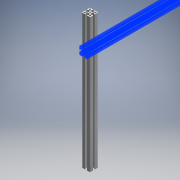
# Autodesk Inventor part: Propile_500
Saved by Autodesk Inventor 2019 (Build 230136000, 136)
## iProperties
Created: 2019-04-24
Part Number: Propile_500
Material: 알루미늄 6061
Document SubType Name: Modeling
Designer: hinmo
Density: 2.7 g/cm^3
Appearance: 알루미늄 - 평지
Mass: 433.812 g
Surface Area: 1856.02 cm^2
Volume: 160.671 cm^3
Author: hinmo
Autodesk Inventor part; units mm, degrees
ref_plane "YZ Plane" through (0, 0, 0) normal (1, 0, 0) x (0, 1, 0)
ref_plane "XZ Plane" through (0, 0, 0) normal (0, 1, 0) x (-1, 0, 0)
ref_plane "XY Plane" through (0, 0, 0) normal (0, 0, 1) x (1, 0, 0)
sketch "스케치1" plane through (0, 0, 0) normal (0, 1, 0) x (-1, 0, 0)
  arc A0 (556.3252, 935.7031) -> (557.3252, 936.7031) centre (556.3252, 936.7031) ccw projected
  line L0 (557.3252, 936.7031) -> (557.3252, 938.2031) projected
  line L1 (557.3252, 938.2031) -> (555.3752, 938.2031) projected
  line L2 (555.3752, 938.2031) -> (554.3965, 941.8963) projected
  arc A1 (557.0402, 946.2031) -> (554.3965, 941.8963) centre (561.0724, 940.7632) ccw projected
  line L3 (557.0402, 946.2031) -> (559.9752, 946.2031) projected
  line L4 (559.9752, 946.2031) -> (560.4752, 946.7031) projected
  line L5 (560.4752, 946.7031) -> (560.9752, 946.2031) projected
  line L6 (560.9752, 946.2031) -> (563.9102, 946.2031) projected
  arc A2 (566.5539, 941.8963) -> (563.9102, 946.2031) centre (559.878, 940.7632) ccw projected
  line L7 (566.5539, 941.8963) -> (565.5752, 938.2031) projected
  line L8 (565.5752, 938.2031) -> (563.6252, 938.2031) projected
  line L9 (563.6252, 938.2031) -> (563.6252, 936.7031) projected
  arc A3 (563.6252, 936.7031) -> (564.6252, 935.7031) centre (564.6252, 936.7031) ccw projected
  line L10 (564.6252, 935.7031) -> (573.9752, 935.7031) projected
  arc A4 (573.9752, 935.7031) -> (575.4752, 937.2031) centre (573.9752, 937.2031) ccw projected
  line L11 (575.4752, 937.2031) -> (575.4752, 946.5531) projected
  arc A5 (575.4752, 946.5531) -> (574.4752, 947.5531) centre (574.4752, 946.5531) ccw projected
  line L12 (574.4752, 947.5531) -> (572.9752, 947.5531) projected
  line L13 (572.9752, 947.5531) -> (572.9752, 945.6031) projected
  line L14 (572.9752, 945.6031) -> (569.282, 944.6244) projected
  arc A6 (564.9752, 947.2681) -> (569.282, 944.6244) centre (570.4151, 951.3003) ccw projected
  line L15 (564.9752, 947.2681) -> (564.9752, 950.2031) projected
  line L16 (564.9752, 950.2031) -> (564.4752, 950.7031) projected
  line L17 (564.4752, 950.7031) -> (564.9752, 951.2031) projected
  line L18 (564.9752, 951.2031) -> (564.9752, 954.1381) projected
  arc A7 (569.282, 956.7818) -> (564.9752, 954.1381) centre (570.4151, 950.1059) ccw projected
  line L19 (569.282, 956.7818) -> (572.9752, 955.8031) projected
  line L20 (572.9752, 955.8031) -> (572.9752, 953.8531) projected
  line L21 (572.9752, 953.8531) -> (574.4752, 953.8531) projected
  arc A8 (574.4752, 953.8531) -> (575.4752, 954.8531) centre (574.4752, 954.8531) ccw projected
  line L22 (575.4752, 954.8531) -> (575.4752, 964.2031) projected
  arc A9 (575.4752, 964.2031) -> (573.9752, 965.7031) centre (573.9752, 964.2031) ccw projected
  line L23 (573.9752, 965.7031) -> (564.6252, 965.7031) projected
  arc A10 (564.6252, 965.7031) -> (563.6252, 964.7031) centre (564.6252, 964.7031) ccw projected
  line L24 (563.6252, 964.7031) -> (563.6252, 963.2031) projected
  line L25 (563.6252, 963.2031) -> (565.5752, 963.2031) projected
  line L26 (565.5752, 963.2031) -> (566.5539, 959.51) projected
  arc A11 (563.9102, 955.2031) -> (566.5539, 959.51) centre (559.878, 960.6431) ccw projected
  line L27 (563.9102, 955.2031) -> (560.9752, 955.2031) projected
  line L28 (560.9752, 955.2031) -> (560.4752, 954.7031) projected
  line L29 (560.4752, 954.7031) -> (559.9752, 955.2031) projected
  line L30 (559.9752, 955.2031) -> (557.0402, 955.2031) projected
  arc A12 (554.3965, 959.51) -> (557.0402, 955.2031) centre (561.0724, 960.6431) ccw projected
  line L31 (554.3965, 959.51) -> (555.3752, 963.2031) projected
  line L32 (555.3752, 963.2031) -> (557.3252, 963.2031) projected
  line L33 (557.3252, 963.2031) -> (557.3252, 964.7031) projected
  arc A13 (557.3252, 964.7031) -> (556.3252, 965.7031) centre (556.3252, 964.7031) ccw projected
  line L34 (556.3252, 965.7031) -> (546.9752, 965.7031) projected
  arc A14 (546.9752, 965.7031) -> (545.4752, 964.2031) centre (546.9752, 964.2031) ccw projected
  line L35 (545.4752, 964.2031) -> (545.4752, 954.8531) projected
  arc A15 (545.4752, 954.8531) -> (546.4752, 953.8531) centre (546.4752, 954.8531) ccw projected
  line L36 (546.4752, 953.8531) -> (547.9752, 953.8531) projected
  line L37 (547.9752, 953.8531) -> (547.9752, 955.8031) projected
  line L38 (547.9752, 955.8031) -> (551.6683, 956.7818) projected
  arc A16 (555.9752, 954.1381) -> (551.6683, 956.7818) centre (550.5352, 950.1059) ccw projected
  line L39 (555.9752, 954.1381) -> (555.9752, 951.2031) projected
  line L40 (555.9752, 951.2031) -> (556.4752, 950.7031) projected
  line L41 (556.4752, 950.7031) -> (555.9752, 950.2031) projected
  line L42 (555.9752, 950.2031) -> (555.9752, 947.2681) projected
  arc A17 (551.6683, 944.6244) -> (555.9752, 947.2681) centre (550.5352, 951.3003) ccw projected
  line L43 (551.6683, 944.6244) -> (547.9752, 945.6031) projected
  line L44 (547.9752, 945.6031) -> (547.9752, 947.5531) projected
  line L45 (547.9752, 947.5531) -> (546.4752, 947.5531) projected
  arc A18 (546.4752, 947.5531) -> (545.4752, 946.5531) centre (546.4752, 946.5531) ccw projected
  line L46 (545.4752, 946.5531) -> (545.4752, 937.2031) projected
  arc A19 (545.4752, 937.2031) -> (546.9752, 935.7031) centre (546.9752, 937.2031) ccw projected
  line L47 (546.9752, 935.7031) -> (556.3252, 935.7031) projected
  arc A20 (573.0595, 959.1795) -> (573.0595, 962.2268) centre (570.4752, 960.7031) ccw projected
  line L48 (573.0595, 959.1795) -> (574.0055, 958.2335) projected
  line L49 (574.0055, 958.2335) -> (572.9448, 957.1728) projected
  line L50 (572.9448, 957.1728) -> (571.9988, 958.1188) projected
  arc A21 (568.9515, 958.1188) -> (571.9988, 958.1188) centre (570.4752, 960.7031) ccw projected
  line L51 (568.9515, 958.1188) -> (568.0055, 957.1728) projected
  line L52 (568.0055, 957.1728) -> (566.9448, 958.2335) projected
  line L53 (566.9448, 958.2335) -> (567.8909, 959.1795) projected
  arc A22 (567.8909, 962.2268) -> (567.8909, 959.1795) centre (570.4752, 960.7031) ccw projected
  line L54 (567.8909, 962.2268) -> (566.9448, 963.1728) projected
  line L55 (566.9448, 963.1728) -> (568.0055, 964.2335) projected
  line L56 (568.0055, 964.2335) -> (568.9515, 963.2874) projected
  arc A23 (571.9988, 963.2874) -> (568.9515, 963.2874) centre (570.4752, 960.7031) ccw projected
  line L57 (571.9988, 963.2874) -> (572.9448, 964.2335) projected
  line L58 (572.9448, 964.2335) -> (574.0055, 963.1728) projected
  line L59 (574.0055, 963.1728) -> (573.0595, 962.2268) projected
  line L60 (563.5055, 952.6728) -> (562.5713, 952.0656) projected
  arc A24 (562.5713, 949.3407) -> (562.5713, 952.0656) centre (560.4752, 950.7031) ccw projected
  line L61 (562.5713, 949.3407) -> (563.5055, 948.7335) projected
  line L62 (563.5055, 948.7335) -> (562.4448, 947.6728) projected
  line L63 (562.4448, 947.6728) -> (561.8376, 948.607) projected
  arc A25 (559.1127, 948.607) -> (561.8376, 948.607) centre (560.4752, 950.7031) ccw projected
  line L64 (559.1127, 948.607) -> (558.5055, 947.6728) projected
  line L65 (558.5055, 947.6728) -> (557.4448, 948.7335) projected
  line L66 (557.4448, 948.7335) -> (558.3791, 949.3407) projected
  arc A26 (558.3791, 952.0656) -> (558.3791, 949.3407) centre (560.4752, 950.7031) ccw projected
  line L67 (558.3791, 952.0656) -> (557.4448, 952.6728) projected
  line L68 (557.4448, 952.6728) -> (558.5055, 953.7335) projected
  line L69 (558.5055, 953.7335) -> (559.1127, 952.7992) projected
  arc A27 (561.8376, 952.7992) -> (559.1127, 952.7992) centre (560.4752, 950.7031) ccw projected
  line L70 (561.8376, 952.7992) -> (562.4448, 953.7335) projected
  line L71 (562.4448, 953.7335) -> (563.5055, 952.6728) projected
  arc A28 (571.9988, 943.2874) -> (568.9515, 943.2874) centre (570.4752, 940.7031) ccw projected
  line L72 (571.9988, 943.2874) -> (572.9448, 944.2335) projected
  line L73 (572.9448, 944.2335) -> (574.0055, 943.1728) projected
  line L74 (574.0055, 943.1728) -> (573.0595, 942.2268) projected
  arc A29 (573.0595, 939.1795) -> (573.0595, 942.2268) centre (570.4752, 940.7031) ccw projected
  line L75 (573.0595, 939.1795) -> (574.0055, 938.2335) projected
  line L76 (574.0055, 938.2335) -> (572.9448, 937.1728) projected
  line L77 (572.9448, 937.1728) -> (571.9988, 938.1188) projected
  arc A30 (568.9515, 938.1188) -> (571.9988, 938.1188) centre (570.4752, 940.7031) ccw projected
  line L78 (568.9515, 938.1188) -> (568.0055, 937.1728) projected
  line L79 (568.0055, 937.1728) -> (566.9448, 938.2335) projected
  line L80 (566.9448, 938.2335) -> (567.8909, 939.1795) projected
  arc A31 (567.8909, 942.2268) -> (567.8909, 939.1795) centre (570.4752, 940.7031) ccw projected
  line L81 (567.8909, 942.2268) -> (566.9448, 943.1728) projected
  line L82 (566.9448, 943.1728) -> (568.0055, 944.2335) projected
  line L83 (568.0055, 944.2335) -> (568.9515, 943.2874) projected
  arc A32 (548.9515, 958.1188) -> (551.9988, 958.1188) centre (550.4752, 960.7031) ccw projected
  line L84 (548.9515, 958.1188) -> (548.0055, 957.1728) projected
  line L85 (548.0055, 957.1728) -> (546.9448, 958.2335) projected
  line L86 (546.9448, 958.2335) -> (547.8909, 959.1795) projected
  arc A33 (547.8909, 962.2268) -> (547.8909, 959.1795) centre (550.4752, 960.7031) ccw projected
  line L87 (547.8909, 962.2268) -> (546.9448, 963.1728) projected
  line L88 (546.9448, 963.1728) -> (548.0055, 964.2335) projected
  line L89 (548.0055, 964.2335) -> (548.9515, 963.2874) projected
  arc A34 (551.9988, 963.2874) -> (548.9515, 963.2874) centre (550.4752, 960.7031) ccw projected
  line L90 (551.9988, 963.2874) -> (552.9448, 964.2335) projected
  line L91 (552.9448, 964.2335) -> (554.0055, 963.1728) projected
  line L92 (554.0055, 963.1728) -> (553.0595, 962.2268) projected
  arc A35 (553.0595, 959.1795) -> (553.0595, 962.2268) centre (550.4752, 960.7031) ccw projected
  line L93 (553.0595, 959.1795) -> (554.0055, 958.2335) projected
  line L94 (554.0055, 958.2335) -> (552.9448, 957.1728) projected
  line L95 (552.9448, 957.1728) -> (551.9988, 958.1188) projected
  arc A36 (553.0595, 939.1795) -> (553.0595, 942.2268) centre (550.4752, 940.7031) ccw projected
  line L96 (553.0595, 939.1795) -> (554.0055, 938.2335) projected
  line L97 (554.0055, 938.2335) -> (552.9448, 937.1728) projected
  line L98 (552.9448, 937.1728) -> (551.9988, 938.1188) projected
  arc A37 (548.9515, 938.1188) -> (551.9988, 938.1188) centre (550.4752, 940.7031) ccw projected
  line L99 (548.9515, 938.1188) -> (548.0055, 937.1728) projected
  line L100 (548.0055, 937.1728) -> (546.9448, 938.2335) projected
  line L101 (546.9448, 938.2335) -> (547.8909, 939.1795) projected
  arc A38 (547.8909, 942.2268) -> (547.8909, 939.1795) centre (550.4752, 940.7031) ccw projected
  line L102 (547.8909, 942.2268) -> (546.9448, 943.1728) projected
  line L103 (546.9448, 943.1728) -> (548.0055, 944.2335) projected
  line L104 (548.0055, 944.2335) -> (548.9515, 943.2874) projected
  arc A39 (551.9988, 943.2874) -> (548.9515, 943.2874) centre (550.4752, 940.7031) ccw projected
  line L105 (551.9988, 943.2874) -> (552.9448, 944.2335) projected
  line L106 (552.9448, 944.2335) -> (554.0055, 943.1728) projected
  line L107 (554.0055, 943.1728) -> (553.0595, 942.2268) projected
  arc A40 (-4.15, -15) -> (-3.15, -14) centre (-4.15, -14) ccw
  line L108 (-3.15, -14) -> (-3.15, -12.5)
  line L109 (-3.15, -12.5) -> (-5.1, -12.5)
  line L110 (-5.1, -12.5) -> (-6.0787, -8.8068)
  arc A41 (-3.435, -4.5) -> (-6.0787, -8.8068) centre (0.5972, -9.94) ccw
  line L111 (-3.435, -4.5) -> (-0.5, -4.5)
  line L112 (-0.5, -4.5) -> (0, -4)
  line L113 (0, -4) -> (0.5, -4.5)
  line L114 (0.5, -4.5) -> (3.435, -4.5)
  arc A42 (6.0787, -8.8068) -> (3.435, -4.5) centre (-0.5972, -9.94) ccw
  line L115 (6.0787, -8.8068) -> (5.1, -12.5)
  line L116 (5.1, -12.5) -> (3.15, -12.5)
  line L117 (3.15, -12.5) -> (3.15, -14)
  arc A43 (3.15, -14) -> (4.15, -15) centre (4.15, -14) ccw
  line L118 (4.15, -15) -> (13.5, -15)
  arc A44 (13.5, -15) -> (15, -13.5) centre (13.5, -13.5) ccw
  line L119 (15, -13.5) -> (15, -4.15)
  arc A45 (15, -4.15) -> (14, -3.15) centre (14, -4.15) ccw
  line L120 (14, -3.15) -> (12.5, -3.15)
  line L121 (12.5, -3.15) -> (12.5, -5.1)
  line L122 (12.5, -5.1) -> (8.8068, -6.0787)
  arc A46 (4.5, -3.435) -> (8.8068, -6.0787) centre (9.94, 0.5972) ccw
  line L123 (4.5, -3.435) -> (4.5, -0.5)
  line L124 (4.5, -0.5) -> (4, 0)
  line L125 (4, 0) -> (4.5, 0.5)
  line L126 (4.5, 0.5) -> (4.5, 3.435)
  arc A47 (8.8068, 6.0787) -> (4.5, 3.435) centre (9.94, -0.5972) ccw
  line L127 (8.8068, 6.0787) -> (12.5, 5.1)
  line L128 (12.5, 5.1) -> (12.5, 3.15)
  line L129 (12.5, 3.15) -> (14, 3.15)
  arc A48 (14, 3.15) -> (15, 4.15) centre (14, 4.15) ccw
  line L130 (15, 4.15) -> (15, 13.5)
  arc A49 (15, 13.5) -> (13.5, 15) centre (13.5, 13.5) ccw
  line L131 (13.5, 15) -> (4.15, 15)
  arc A50 (4.15, 15) -> (3.15, 14) centre (4.15, 14) ccw
  line L132 (3.15, 14) -> (3.15, 12.5)
  line L133 (3.15, 12.5) -> (5.1, 12.5)
  line L134 (5.1, 12.5) -> (6.0787, 8.8068)
  arc A51 (3.435, 4.5) -> (6.0787, 8.8068) centre (-0.5972, 9.94) ccw
  line L135 (3.435, 4.5) -> (0.5, 4.5)
  line L136 (0.5, 4.5) -> (0, 4)
  line L137 (0, 4) -> (-0.5, 4.5)
  line L138 (-0.5, 4.5) -> (-3.435, 4.5)
  arc A52 (-6.0787, 8.8068) -> (-3.435, 4.5) centre (0.5972, 9.94) ccw
  line L139 (-6.0787, 8.8068) -> (-5.1, 12.5)
  line L140 (-5.1, 12.5) -> (-3.15, 12.5)
  line L141 (-3.15, 12.5) -> (-3.15, 14)
  arc A53 (-3.15, 14) -> (-4.15, 15) centre (-4.15, 14) ccw
  line L142 (-4.15, 15) -> (-13.5, 15)
  arc A54 (-13.5, 15) -> (-15, 13.5) centre (-13.5, 13.5) ccw
  line L143 (-15, 13.5) -> (-15, 4.15)
  arc A55 (-15, 4.15) -> (-14, 3.15) centre (-14, 4.15) ccw
  line L144 (-14, 3.15) -> (-12.5, 3.15)
  line L145 (-12.5, 3.15) -> (-12.5, 5.1)
  line L146 (-12.5, 5.1) -> (-8.8068, 6.0787)
  arc A56 (-4.5, 3.435) -> (-8.8068, 6.0787) centre (-9.94, -0.5972) ccw
  line L147 (-4.5, 3.435) -> (-4.5, 0.5)
  line L148 (-4.5, 0.5) -> (-4, 0)
  line L149 (-4, 0) -> (-4.5, -0.5)
  line L150 (-4.5, -0.5) -> (-4.5, -3.435)
  arc A57 (-8.8068, -6.0787) -> (-4.5, -3.435) centre (-9.94, 0.5972) ccw
  line L151 (-8.8068, -6.0787) -> (-12.5, -5.1)
  line L152 (-12.5, -5.1) -> (-12.5, -3.15)
  line L153 (-12.5, -3.15) -> (-14, -3.15)
  arc A58 (-14, -3.15) -> (-15, -4.15) centre (-14, -4.15) ccw
  line L154 (-15, -4.15) -> (-15, -13.5)
  arc A59 (-15, -13.5) -> (-13.5, -15) centre (-13.5, -13.5) ccw
  line L155 (-13.5, -15) -> (-4.15, -15)
  arc A60 (12.5843, 8.4764) -> (12.5843, 11.5236) centre (10, 10) ccw
  line L156 (12.5843, 8.4764) -> (13.5303, 7.5303)
  line L157 (13.5303, 7.5303) -> (12.4697, 6.4697)
  line L158 (12.4697, 6.4697) -> (11.5236, 7.4157)
  arc A61 (8.4764, 7.4157) -> (11.5236, 7.4157) centre (10, 10) ccw
  line L159 (8.4764, 7.4157) -> (7.5303, 6.4697)
  line L160 (7.5303, 6.4697) -> (6.4697, 7.5303)
  line L161 (6.4697, 7.5303) -> (7.4157, 8.4764)
  arc A62 (7.4157, 11.5236) -> (7.4157, 8.4764) centre (10, 10) ccw
  line L162 (7.4157, 11.5236) -> (6.4697, 12.4697)
  line L163 (6.4697, 12.4697) -> (7.5303, 13.5303)
  line L164 (7.5303, 13.5303) -> (8.4764, 12.5843)
  arc A63 (11.5236, 12.5843) -> (8.4764, 12.5843) centre (10, 10) ccw
  line L165 (11.5236, 12.5843) -> (12.4697, 13.5303)
  line L166 (12.4697, 13.5303) -> (13.5303, 12.4697)
  line L167 (13.5303, 12.4697) -> (12.5843, 11.5236)
  line L168 (3.0303, 1.9697) -> (2.0961, 1.3624)
  arc A64 (2.0961, -1.3624) -> (2.0961, 1.3624) centre (0, 0) ccw
  line L169 (2.0961, -1.3624) -> (3.0303, -1.9697)
  line L170 (3.0303, -1.9697) -> (1.9697, -3.0303)
  line L171 (1.9697, -3.0303) -> (1.3624, -2.0961)
  arc A65 (-1.3624, -2.0961) -> (1.3624, -2.0961) centre (0, 0) ccw
  line L172 (-1.3624, -2.0961) -> (-1.9697, -3.0303)
  line L173 (-1.9697, -3.0303) -> (-3.0303, -1.9697)
  line L174 (-3.0303, -1.9697) -> (-2.0961, -1.3624)
  arc A66 (-2.0961, 1.3624) -> (-2.0961, -1.3624) centre (0, 0) ccw
  line L175 (-2.0961, 1.3624) -> (-3.0303, 1.9697)
  line L176 (-3.0303, 1.9697) -> (-1.9697, 3.0303)
  line L177 (-1.9697, 3.0303) -> (-1.3624, 2.0961)
  arc A67 (1.3624, 2.0961) -> (-1.3624, 2.0961) centre (0, 0) ccw
  line L178 (1.3624, 2.0961) -> (1.9697, 3.0303)
  line L179 (1.9697, 3.0303) -> (3.0303, 1.9697)
  arc A68 (11.5236, -7.4157) -> (8.4764, -7.4157) centre (10, -10) ccw
  line L180 (11.5236, -7.4157) -> (12.4697, -6.4697)
  line L181 (12.4697, -6.4697) -> (13.5303, -7.5303)
  line L182 (13.5303, -7.5303) -> (12.5843, -8.4764)
  arc A69 (12.5843, -11.5236) -> (12.5843, -8.4764) centre (10, -10) ccw
  line L183 (12.5843, -11.5236) -> (13.5303, -12.4697)
  line L184 (13.5303, -12.4697) -> (12.4697, -13.5303)
  line L185 (12.4697, -13.5303) -> (11.5236, -12.5843)
  arc A70 (8.4764, -12.5843) -> (11.5236, -12.5843) centre (10, -10) ccw
  line L186 (8.4764, -12.5843) -> (7.5303, -13.5303)
  line L187 (7.5303, -13.5303) -> (6.4697, -12.4697)
  line L188 (6.4697, -12.4697) -> (7.4157, -11.5236)
  arc A71 (7.4157, -8.4764) -> (7.4157, -11.5236) centre (10, -10) ccw
  line L189 (7.4157, -8.4764) -> (6.4697, -7.5303)
  line L190 (6.4697, -7.5303) -> (7.5303, -6.4697)
  line L191 (7.5303, -6.4697) -> (8.4764, -7.4157)
  arc A72 (-11.5236, 7.4157) -> (-8.4764, 7.4157) centre (-10, 10) ccw
  line L192 (-11.5236, 7.4157) -> (-12.4697, 6.4697)
  line L193 (-12.4697, 6.4697) -> (-13.5303, 7.5303)
  line L194 (-13.5303, 7.5303) -> (-12.5843, 8.4764)
  arc A73 (-12.5843, 11.5236) -> (-12.5843, 8.4764) centre (-10, 10) ccw
  line L195 (-12.5843, 11.5236) -> (-13.5303, 12.4697)
  line L196 (-13.5303, 12.4697) -> (-12.4697, 13.5303)
  line L197 (-12.4697, 13.5303) -> (-11.5236, 12.5843)
  arc A74 (-8.4764, 12.5843) -> (-11.5236, 12.5843) centre (-10, 10) ccw
  line L198 (-8.4764, 12.5843) -> (-7.5303, 13.5303)
  line L199 (-7.5303, 13.5303) -> (-6.4697, 12.4697)
  line L200 (-6.4697, 12.4697) -> (-7.4157, 11.5236)
  arc A75 (-7.4157, 8.4764) -> (-7.4157, 11.5236) centre (-10, 10) ccw
  line L201 (-7.4157, 8.4764) -> (-6.4697, 7.5303)
  line L202 (-6.4697, 7.5303) -> (-7.5303, 6.4697)
  line L203 (-7.5303, 6.4697) -> (-8.4764, 7.4157)
  arc A76 (-7.4157, -11.5236) -> (-7.4157, -8.4764) centre (-10, -10) ccw
  line L204 (-7.4157, -11.5236) -> (-6.4697, -12.4697)
  line L205 (-6.4697, -12.4697) -> (-7.5303, -13.5303)
  line L206 (-7.5303, -13.5303) -> (-8.4764, -12.5843)
  arc A77 (-11.5236, -12.5843) -> (-8.4764, -12.5843) centre (-10, -10) ccw
  line L207 (-11.5236, -12.5843) -> (-12.4697, -13.5303)
  line L208 (-12.4697, -13.5303) -> (-13.5303, -12.4697)
  line L209 (-13.5303, -12.4697) -> (-12.5843, -11.5236)
  arc A78 (-12.5843, -8.4764) -> (-12.5843, -11.5236) centre (-10, -10) ccw
  line L210 (-12.5843, -8.4764) -> (-13.5303, -7.5303)
  line L211 (-13.5303, -7.5303) -> (-12.4697, -6.4697)
  line L212 (-12.4697, -6.4697) -> (-11.5236, -7.4157)
  arc A79 (-8.4764, -7.4157) -> (-11.5236, -7.4157) centre (-10, -10) ccw
  line L213 (-8.4764, -7.4157) -> (-7.5303, -6.4697)
  line L214 (-7.5303, -6.4697) -> (-6.4697, -7.5303)
  line L215 (-6.4697, -7.5303) -> (-7.4157, -8.4764)
  constraints: 216 end point, 80 point on circle, 40 centre point
extrude "돌출1" add sketch "스케치1" along normal blind 500 contours L155 A59 L154 A58 L153 L152 L151 A57 L150 L149 L148 L147 A56 L146 L145 L144 A55 L143 A54 L142 A53 L141 L140 L139 A52 L138 L137 L136 L135 A51 L134 L133 L132 A50 L131 A49 L130 A48 L129 L128 L127 A47 L126 L125 L124 L123 A46 L122 L121 L120 A45 L119 A44 L118 A43 L117 L116 L115 A42 L114 L113 L112 L111 A41 L110 L109 L108 A40
